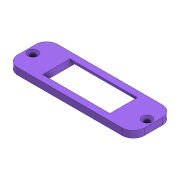
# Autodesk Inventor part: Wago2Din_1Way
Saved by Autodesk Inventor 2021 (Build 250183000, 183)
## iProperties
Created: 2021-07-31
Part Number: Wago2Din_1Way
Material: Generisch
Document SubType Name: Modeling
Designer: Rama
Density: 1 g/cm^3
Appearance: Violett
Author: Rama
Autodesk Inventor part; units mm, degrees
ref_plane "YZ Plane" through (0, 0, 0) normal (1, 0, 0) x (0, 1, 0)
ref_plane "XZ Plane" through (0, 0, 0) normal (0, 1, 0) x (-1, 0, 0)
ref_plane "XY Plane" through (0, 0, 0) normal (0, 0, 1) x (1, 0, 0)
sketch "Skizze1" plane through (0, 0, 0) normal (0, 1, 0) x (-1, 0, 0)
  line L0 (15.1, 6.15) -> (-15.1, 6.15)
  line L1 (-15.1, 6.15) -> (-15.1, -6.15)
  line L2 (-15.1, -6.15) -> (15.1, -6.15)
  line L3 (15.1, -6.15) -> (15.1, 6.15)
  line L4 (15.1, 6.15) -> (-15.1, -6.15) construction
  line L5 (-15.1, 6.15) -> (15.1, -6.15) construction
  line L6 (28.45, 9) -> (-28.45, 9)
  line L7 (-28.45, 9) -> (-28.45, -9)
  line L8 (-28.45, -9) -> (28.45, -9)
  line L9 (28.45, -9) -> (28.45, 9)
  line L10 (28.45, 9) -> (-28.45, -9) construction
  line L11 (-28.45, 9) -> (28.45, -9) construction
  point P0 (0, 0)
  dimension "d0" = 30.2
  dimension "d1" = 12.3
  dimension "d2" = 56.9
  dimension "d3" = 18
  constraints: 24 end point, 4 midpoint, 4 parallel, 2 horizontal, 2 perpendicular
  measures "d0" distance of L2.end L1.end
  measures "d1" distance of L1.end L0.end
  measures "d2" distance of L8.end L7.end
  measures "d3" distance of L7.end L6.end
extrude "Extrusion1" add sketch "Skizze1" along normal blind 3
chamfer "Fase1" distance 2 angle 45 2 edges at (0, 0, -6.15) (0, 0, 6.15)
sketch "Skizze2" plane through (0, 3, 0) normal (0, 1, 0) x (1, 0, 0)
  line L0 (0, 0) -> (-25.65, 0)
  line L1 (-25.65, 0) -> (25.65, 0)
  dimension "d9" = 25.65
  dimension "d10" = 51.3
  constraints: 4 end point, 1 horizontal, 1 point on line
  measures "d9" distance of L0.start L0.end
  measures "d10" distance of L0.end L1.end
hole "Bohrung1" at (25.65, 3, 0) at (-25.65, 3, 0) direction (0, -1, 0) diameter 2.4 end through all countersink diameter 4.4 countersink angle 90 clearance for "Flachkopfmaschinenschraube" size "M2" standard "ANSI Metrisches M Profil"
fillet "Rundung1" radius 5 4 edges at (28.45, 1.5, -9) (28.45, 1.5, 9) (-28.45, 1.5, -9) (-28.45, 1.5, 9)
